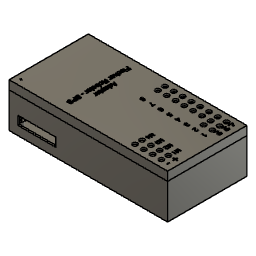
Fischer Technik v16 (Autodesk Fusion 360 design; units mm, degrees)
Autodesk Fusion 360 part; units mm, degrees
sketch "Skizze1" plane through (0, 0, 0) normal (0, 1, 0) x (1, 0, 0)
  line L0 (0, 0) -> (180, 0)
  line L1 (180, 0) -> (180, 90)
  line L2 (180, 90) -> (0, 90)
  line L3 (0, 90) -> (0, 0)
  constraint horizontal L0
  constraint vertical L1
  constraint horizontal L2
  constraint vertical L3
  constraint coincident L0.start L3.end
extrude "Extrusion1" add sketch "Skizze1" along normal blind 30 makes body 1
extrude "Extrusion2" add 1 faces at (60, 30, -60) along direction (0, 1, 0) blind 20 on bodies 1 bodies 1
ref_plane "Arbeitsebene1" through (90, 40, -45) normal (0, 1, 0) x (0, 0, 1)
split "Teilen1" by plane through (90, 40, -45) normal (0, 1, 0) bodies 1 makes body 2 at (60, 50, -60)
shell "Schale1" thickness 2 removed faces 1 at (120, 40, -60) on bodies 1
shell "Schale2" thickness 2 removed faces 1 at (120, 40, -60) on bodies 2
sketch "Skizze4" plane through (0, 0, 0) normal (0, 1, 0) x (1, 0, 0)
  circle A0 centre (6.4995, 82.5) radius 3
  circle A1 centre (172.0121, 7) radius 3
  circle A2 centre (171.9995, 82.5) radius 3
  circle A3 centre (6.5121, 7) radius 3
  dimension "d11" = 6
  dimension "d12" = 6
  dimension "d13" = 6
  dimension "d14" = 6
  dimension "d117" = 165.5
  dimension "d118" = 165.5
  dimension "d119" = 75.5
  dimension "d120" = 75.5
  measures "d11" diameter of A0
  measures "d12" diameter of A1
  measures "d13" diameter of A2
  measures "d14" diameter of A3
  measures "d117" horizontal distance of A0.centre A2.centre
  measures "d118" distance of A1.centre A3.centre
  measures "d119" vertical distance of A0.centre A3.centre
  measures "d120" vertical distance of A1.centre A2.centre
extrude "Extrusion4" add sketch "Skizze4" along normal blind 10 separate body contours A3 makes body 3
extrude "Extrusion5" add sketch "Skizze4" along normal blind 10 separate body contours A1 makes body 4
extrude "Extrusion6" add sketch "Skizze4" along normal blind 10 separate body contours A0 makes body 5
extrude "Extrusion7" add sketch "Skizze4" along normal blind 10 separate body contours A2 makes body 6
sketch "Skizze6" plane through (0, 0, 0) normal (-1, 0, 0) x (0, 0, 1)
  line L0 (0, 40) -> (-90, 40)
  line L1 (-90, 40) -> (-90, 0)
  line L2 (-90, 0) -> (0, 0)
  line L3 (0, 0) -> (0, 40)
  line L4 (-79.5, 20) -> (-10.5, 20)
  line L5 (-10.5, 20) -> (-10.5, 10.0586)
  line L6 (-10.5, 10.0586) -> (-79.5, 10.0586)
  line L7 (-79.5, 10.0586) -> (-79.5, 20)
  dimension "d24" = 69
  constraint horizontal L4
  constraint vertical L5
  constraint horizontal L6
  constraint vertical L7
  measures "d24" distance of L4.start L4.end
extrude "Extrusion8" cut sketch "Skizze6" against normal blind 2 contours L4 L5 L6 L7 bodies 1
sketch "Skizze7" plane through (0, 0, 0) normal (0, 0, 1) x (1, 0, 0)
  line L0 (180, 40) -> (0, 40)
  line L1 (0, 40) -> (0, 0)
  line L2 (0, 0) -> (180, 0)
  line L3 (180, 0) -> (180, 40)
  line L4 (10, 0) -> (53, 0)
  line L5 (53, 0) -> (53, 20)
  line L6 (53, 20) -> (10, 20)
  line L7 (10, 20) -> (10, 0)
  line L8 (10, 20) -> (53, 20)
  line L9 (53, 20) -> (53, 10)
  line L10 (53, 10) -> (10, 10)
  line L11 (10, 10) -> (10, 20)
  dimension "d27" = 43
  dimension "d123" = 10
  constraint horizontal L4
  constraint vertical L5
  constraint horizontal L6
  constraint vertical L7
  constraint coincident L2 L4.start
  constraint horizontal L8
  constraint vertical L9
  constraint horizontal L10
  constraint vertical L11
  constraint midpoint L5 L9.end
  measures "d27" distance of L4.start L4.end
  measures "d123" distance of L1 L7
sketch "Skizze8" plane through (0, 50, 0) normal (0, 1, 0) x (-1, 0, 0)
  line L0 (0, -90) -> (0, 0)
  line L1 (0, 0) -> (-180, 0)
  line L2 (-180, 0) -> (-180, -90)
  line L3 (-180, -90) -> (0, -90)
  point P0 (-165, -82)
  point P1 (-165, -74)
  point P2 (-165, -66)
  point P3 (-155, -82)
  point P4 (-155, -74)
  point P5 (-155, -66)
  point P6 (-145, -82)
  point P7 (-145, -74)
  point P8 (-135, -82)
  point P9 (-135, -74)
  point P10 (-95, -82)
  point P11 (-125, -82)
  point P12 (-115, -82)
  point P13 (-105, -82)
  point P14 (-95, -74)
  point P15 (-125, -74)
  point P16 (-115, -74)
  point P17 (-105, -74)
  dimension "d30" = 8
  dimension "d31" = 8
  dimension "d32" = 8
  dimension "d33" = 10
  dimension "d34" = 10
  dimension "d35" = 15
  dimension "d37" = 10
  dimension "d38" = 10
  dimension "d39" = 10
  dimension "d40" = 10
  dimension "d41" = 10
  constraint vertical P0 P1
  constraint vertical P1 P2
  constraint vertical P3 P4
  constraint vertical P4 P5
  constraint vertical P6 P7
  constraint vertical P8 P9
  constraint vertical P10 P14
  constraint vertical P11 P15
  constraint vertical P12 P16
  constraint vertical P13 P17
  constraint horizontal P0 P3
  constraint horizontal P6 P8
  constraint horizontal P10 P11
  constraint horizontal P12 P13
  constraint horizontal P1 P4
  constraint horizontal P7 P9
  constraint horizontal P14 P15
  constraint horizontal P16 P17
  constraint horizontal P15 P16
  constraint horizontal P9 P14
  constraint horizontal P4 P7
  constraint horizontal P2 P5
  constraint horizontal P3 P6
  constraint horizontal P8 P10
  constraint horizontal P11 P12
  measures "d30" distance of P0 P1
  measures "d31" distance of P1 P2
  measures "d32" distance of L3 P0
  measures "d33" distance of P0 P3
  measures "d34" distance of P3 P6
  measures "d35" distance of L2 P0
  measures "d37" distance of P6 P8
  measures "d38" distance of P8 P11
  measures "d39" distance of P11 P12
  measures "d40" distance of P12 P13
  measures "d41" distance of P10 P13
sketch "Skizze9" plane through (0, 50, 0) normal (0, 1, 0) x (-1, 0, 0)
  line L0 (0, 0) -> (-180, 0)
  point P0 (-165, -16)
  point P1 (-165, -8)
  point P2 (-155, -16)
  point P3 (-155, -8)
  point P4 (-145, -16)
  point P5 (-145, -8)
  point P6 (-135, -16)
  point P7 (-135, -8)
  point P8 (-165, -66)
  point P9 (-135, -74)
  point P10 (-145, -74)
  point P11 (-155, -66)
  dimension "d42" = 8
  dimension "d43" = 8
  constraint vertical P0 P1
  constraint vertical P2 P3
  constraint vertical P4 P5
  constraint vertical P6 P7
  constraint horizontal P0 P2
  constraint horizontal P4 P6
  constraint horizontal P1 P3
  constraint horizontal P5 P7
  constraint vertical P0 P8
  constraint vertical P6 P9
  constraint vertical P4 P10
  constraint vertical P2 P11
  constraint horizontal P2 P4
  constraint horizontal P1 P7
  measures "d42" distance of P1 L0
  measures "d43" distance of P0 P1
hole "Bohrung1" at (165, 50, -82) at (165, 50, -74) at (165, 50, -66) at (155, 50, -82) at (155, 50, -74) at (155, 50, -66) at (165, 50, -16) at (165, 50, -8) at (155, 50, -16) at (155, 50, -8) at (145, 50, -8) at (145, 50, -16) at (135, 50, -16) at (135, 50, -8) at (145, 50, -82) at (145, 50, -74) at (135, 50, -82) at (135, 50, -74) at (125, 50, -82) at (125, 50, -74) at (115, 50, -82) at (105, 50, -82) at (95, 50, -82) at (115, 50, -74) at (105, 50, -74) at (95, 50, -74) direction (0, -1, 0) diameter 5.5 depth 2 tip angle 180 bodies 2
sketch "Skizze10" plane through (0, 50, 0) normal (0, 1, 0) x (-1, 0, 0)
  circle A0 centre (-105, -74) radius 2.75
  circle A1 centre (-95, -82) radius 2.75
  circle A2 centre (-115, -82) radius 2.75
  circle A3 centre (-125, -82) radius 2.75
  circle A4 centre (-135, -82) radius 2.75
  circle A5 centre (-145, -82) radius 2.75
  circle A6 centre (-135, -16) radius 2.75
  circle A7 centre (-145, -8) radius 2.75
  circle A8 centre (-155, -16) radius 2.75
  circle A9 centre (-165, -16) radius 2.75
  circle A10 centre (-155, -74) radius 2.75
  circle A11 centre (-165, -66) radius 2.75
  circle A12 centre (-165, -82) radius 2.75
  circle A13 centre (-165, -74) radius 2.75
  circle A14 centre (-155, -82) radius 2.75
  circle A15 centre (-155, -66) radius 2.75
  circle A16 centre (-165, -8) radius 2.75
  circle A17 centre (-155, -8) radius 2.75
  circle A18 centre (-145, -16) radius 2.75
  circle A19 centre (-135, -8) radius 2.75
  circle A20 centre (-145, -74) radius 2.75
  circle A21 centre (-135, -74) radius 2.75
  circle A22 centre (-125, -74) radius 2.75
  circle A23 centre (-105, -82) radius 2.75
  circle A24 centre (-115, -74) radius 2.75
  circle A25 centre (-95, -74) radius 2.75
  line L0 (0, -90) -> (0, 0)
  line L1 (0, 0) -> (-180, 0)
  line L2 (-180, 0) -> (-180, -90)
  line L3 (-180, -90) -> (0, -90)
  line L4 (-171.0364, -76.774) -> (-170.9517, -76.7754) construction
  line L5 (-170.9517, -76.7754) -> (-170.8917, -73.1568) construction
  line L6 (-170.8917, -73.1568) -> (-170.9764, -73.1554) construction
  line L7 (-170.9764, -73.1554) -> (-171.0364, -76.774) construction
  line L8 (-171.0447, -69.2672) -> (-170.9608, -69.2686) construction
  line L9 (-170.9608, -69.2686) -> (-170.8838, -64.656) construction
  line L10 (-170.8838, -64.656) -> (-170.9677, -64.6546) construction
  line L11 (-170.9677, -64.6546) -> (-171.0447, -69.2672) construction
  line L12 (-162.4935, -58.9995) -> (-162.4944, -54.6405) construction
  line L13 (-162.4944, -54.6405) -> (-167.5074, -54.6415) construction
  line L14 (-167.5074, -54.6415) -> (-167.5065, -59.0005) construction
  line L15 (-167.5065, -59.0005) -> (-162.4935, -58.9995) construction
  line L16 (-152.495, -59.6156) -> (-152.4933, -54.0295) construction
  line L17 (-152.4933, -54.0295) -> (-157.5033, -54.028) construction
  line L18 (-157.5033, -54.028) -> (-157.505, -59.6141) construction
  line L19 (-157.505, -59.6141) -> (-152.495, -59.6156) construction
  line L20 (-142.5028, -60.1186) -> (-142.4948, -53.5355) construction
  line L21 (-142.4948, -53.5355) -> (-147.4893, -53.5295) construction
  line L22 (-147.4893, -53.5295) -> (-147.4972, -60.1126) construction
  line L23 (-147.4972, -60.1126) -> (-142.5028, -60.1186) construction
  line L24 (-132.5014, -60.1298) -> (-132.5029, -53.51) construction
  line L25 (-132.5029, -53.51) -> (-137.5001, -53.5111) construction
  line L26 (-137.5001, -53.5111) -> (-137.4986, -60.1309) construction
  line L27 (-137.4986, -60.1309) -> (-132.5014, -60.1298) construction
  line L28 (-122.0178, -60.1305) -> (-121.9983, -53.5468) construction
  line L29 (-121.9983, -53.5468) -> (-127.9627, -53.5292) construction
  line L30 (-127.9627, -53.5292) -> (-127.9822, -60.1129) construction
  line L31 (-127.9822, -60.1129) -> (-122.0178, -60.1305) construction
  line L32 (-112.0324, -60.6387) -> (-111.9975, -53.0581) construction
  line L33 (-111.9975, -53.0581) -> (-117.9326, -53.0307) construction
  line L34 (-117.9326, -53.0307) -> (-117.9676, -60.6113) construction
  line L35 (-117.9676, -60.6113) -> (-112.0324, -60.6387) construction
  line L36 (-162.5074, -26.261) -> (-162.5038, -23.0028) construction
  line L37 (-162.5038, -23.0028) -> (-167.4962, -22.9972) construction
  line L38 (-167.4962, -22.9972) -> (-167.4998, -26.2555) construction
  line L39 (-167.4998, -26.2555) -> (-162.5074, -26.261) construction
  line L40 (-142.0105, -27.6502) -> (-142.0044, -21.6148) construction
  line L41 (-142.0044, -21.6148) -> (-147.9956, -21.6087) construction
  line L42 (-147.9956, -21.6087) -> (-148.0018, -27.6441) construction
  line L43 (-148.0018, -27.6441) -> (-142.0105, -27.6502) construction
  line L44 (-151.9984, -29.1437) -> (-151.9995, -20.1075) construction
  line L45 (-151.9995, -20.1075) -> (-158.0005, -20.1083) construction
  line L46 (-158.0005, -20.1083) -> (-157.9994, -29.1445) construction
  line L47 (-157.9994, -29.1445) -> (-151.9984, -29.1437) construction
  line L48 (-132.512, -27.6497) -> (-132.505, -21.6146) construction
  line L49 (-132.505, -21.6146) -> (-137.495, -21.6088) construction
  line L50 (-137.495, -21.6088) -> (-137.502, -27.6439) construction
  line L51 (-137.502, -27.6439) -> (-132.512, -27.6497) construction
  line L52 (-169.8709, -84.3652) -> (-166.7741, -84.3566) construction
  line L53 (-166.7741, -84.3566) -> (-166.7871, -79.6263) construction
  line L54 (-166.7871, -79.6263) -> (-169.884, -79.6348) construction
  line L55 (-169.884, -79.6348) -> (-169.8709, -84.3652) construction
  line L56 (-101.5, -61.8325) -> (-101.5, -51.8096) construction
  line L57 (-101.5, -51.8096) -> (-108.5, -51.8096) construction
  line L58 (-108.5, -51.8096) -> (-108.5, -61.8325) construction
  line L59 (-108.5, -61.8325) -> (-101.5, -61.8325) construction
  line L60 (-92.065, -62.0835) -> (-92.065, -51.5586) construction
  line L61 (-92.065, -51.5586) -> (-97.935, -51.5586) construction
  line L62 (-97.935, -51.5586) -> (-97.935, -62.0835) construction
  line L63 (-97.935, -62.0835) -> (-92.065, -62.0835) construction
  line L64 (-169.7376, -19.25) -> (-169.7376, -12.75) construction
  line L65 (-169.7376, -12.75) -> (-174.2376, -12.75) construction
  line L66 (-174.2376, -12.75) -> (-174.2376, -19.25) construction
  line L67 (-174.2376, -19.25) -> (-169.7376, -19.25) construction
  line L68 (-168.75, -11.2496) -> (-168.75, -4.7504) construction
  line L69 (-168.75, -4.7504) -> (-174.3763, -4.7504) construction
  line L70 (-174.3763, -4.7504) -> (-174.3763, -11.2496) construction
  line L71 (-174.3763, -11.2496) -> (-168.75, -11.2496) construction
  point P0 (-165, -66)
  point P1 (-155, -66)
  point P2 (-145, -74)
  point P3 (-135, -74)
  point P4 (-165, -16)
  point P5 (-155, -16)
  point P6 (-145, -16)
  point P7 (-135, -16)
  point P8 (-165, -8)
  dimension "d48" = 4
  dimension "d49" = 4
  dimension "d50" = 5
  dimension "d51" = 5
  dimension "d52" = 5
  dimension "d53" = 5
  dimension "d54" = 5
  dimension "d55" = 5
  dimension "d60" = 4
  dimension "d61" = 4
  dimension "d62" = 4
  dimension "d63" = 4
  dimension "d65" = 7
  dimension "d66" = 7
  dimension "d110" = 6
  dimension "d111" = 6
  dimension "d124" = 5
  dimension "d127" = 5
  dimension "d128" = 5
  dimension "d129" = 7
  dimension "d130" = 7
  text T0 "9V" font "Arial" height 4 align centre top in box 0.0847 x 3.6191 at (-171.0364, -76.774) x (0.999863, -0.016561) y (0.016561, 0.999863) spacing 1 kerned
  text T1 "0V" font "Arial" height 4 align centre top in box 0.0839 x 4.6133 at (-171.0447, -69.2672) x (0.999861, -0.01669) y (0.01669, 0.999861) spacing 1 kerned
  text T2 "1" font "Arial" height 5 align centre top in box 4.359 x 5.0129 at (-162.4935, -58.9995) x (-0.000209, 1) y (-1, -0.000209) spacing 1 kerned
  text T3 "2" font "Arial" height 5 align centre top in box 5.5861 x 5.01 at (-152.495, -59.6156) x (0.00031, 1) y (-1, 0.00031) spacing 1 kerned
  text T4 "3\n" font "Arial" height 5 align centre top in box 6.5831 x 4.9945 at (-142.5028, -60.1186) x (0.001213, 0.999999) y (-0.999999, 0.001213) spacing 1 kerned
  text T5 "4" font "Arial" height 5 align centre top in box 6.6198 x 4.9972 at (-132.5014, -60.1298) x (-0.000226, 1) y (-1, -0.000226) spacing 1 kerned
  text T6 "5" font "Arial" height 5 align centre top in box 6.5838 x 5.9644 at (-122.0178, -60.1305) x (0.002958, 0.999996) y (-0.999996, 0.002958) spacing 1 kerned
  text T7 "6" font "Arial" height 5 align centre top in box 7.5807 x 5.9352 at (-112.0324, -60.6387) x (0.004609, 0.999989) y (-0.999989, 0.004609) spacing 1 kerned
  text T8 "M1" font "Arial" height 4 align centre top in box 3.2583 x 4.9924 at (-162.5074, -26.261) x (0.001108, 0.999999) y (-0.999999, 0.001108) spacing 1 kerned
  text T9 "M3" font "Arial" height 4 align centre top in box 6.0354 x 5.9913 at (-142.0105, -27.6502) x (0.001018, 0.999999) y (-0.999999, 0.001018) spacing 1 kerned
  text T10 "M2" font "Arial" height 4 align centre top in box 9.0362 x 6.001 at (-151.9984, -29.1437) x (-0.000121, 1) y (-1, -0.000121) spacing 1 kerned
  text T11 "M4" font "Arial" height 4 align centre top in box 6.0351 x 4.99 at (-132.512, -27.6497) x (0.001164, 0.999999) y (-0.999999, 0.001164) spacing 1 kerned
  text T12 "I" font "Arial" height 5 align left top in box 3.0969 x 4.7304 at (-169.8709, -84.3652) x (0.999996, 0.002757) y (-0.002757, 0.999996) spacing 1 kerned
  text T13 "7" font "Arial" height 5 align centre middle in box 10.0229 x 7 at (-101.5, -61.8325) x (0, 1) y (-1, 0) spacing 1 kerned
  text T14 "8" font "Arial" height 5 align centre middle in box 10.5249 x 5.87 at (-92.065, -62.0835) x (0, 1) y (-1, 0) spacing 1 kerned
  text T15 "+" font "Arial" height 7 align centre middle in box 6.5 x 4.5 at (-169.7376, -19.25) x (0, 1) y (-1, 0) spacing 1 kerned
  text T16 "-" font "Arial" height 7 align centre middle in box 6.4992 x 5.6263 at (-168.75, -11.2496) x (0, 1) y (-1, 0) spacing 1 kerned
  constraint vertical P0
  constraint vertical P1
  constraint vertical P2
  constraint vertical P3
  constraint vertical A22.centre
  constraint vertical A24.centre
  constraint vertical P4
  constraint vertical P5
  constraint vertical P6
  constraint vertical P7
  constraint horizontal A12.centre
  constraint vertical A0.centre
  constraint vertical A25.centre
  constraint horizontal P4
  constraint horizontal P8
  measures "d65" distance of P4
  measures "d66" distance of P0
  measures "d110" distance of P0
  measures "d111" distance of A13.centre
combine "Kombinieren1" operation add target body 1 tool bodies 3 4 5 6
hole "Bohrung2" at (6.5121, 10, -7) direction (0, -1, 0) diameter 1.9 depth 7 tip angle 180 bodies 1
hole "Bohrung3" at (6.4995, 10, -82.5) direction (0, -1, 0) diameter 1.9 depth 7 tip angle 180 bodies 1
hole "Bohrung4" at (171.9995, 10, -82.5) direction (0, -1, 0) diameter 1.9 depth 7 tip angle 180 bodies 1
hole "Bohrung5" at (172.0121, 10, -7) direction (0, -1, 0) diameter 1.9 depth 7 tip angle 180 bodies 1
extrude "Extrusion12" cut sketch "Skizze7" against normal blind 1 contours L5 L6 L7 L8 L9 L10 L11 bodies 1
sketch "Skizze11" plane through (0, 50, 0) normal (0, 1, 0) x (-1, 0, 0)
  line L0 (0, -90) -> (0, 0)
  line L1 (0, 0) -> (-180, 0)
  line L2 (-180, 0) -> (-180, -90)
  line L3 (-180, -90) -> (0, -90)
  circle A0 centre (-95, -74) radius 2.75
  circle A1 centre (-115, -74) radius 2.75
  circle A2 centre (-105, -82) radius 2.75
  circle A3 centre (-125, -74) radius 2.75
  circle A4 centre (-135, -74) radius 2.75
  circle A5 centre (-145, -74) radius 2.75
  circle A6 centre (-135, -8) radius 2.75
  circle A7 centre (-145, -16) radius 2.75
  circle A8 centre (-155, -8) radius 2.75
  circle A9 centre (-165, -8) radius 2.75
  circle A10 centre (-155, -66) radius 2.75
  circle A11 centre (-155, -82) radius 2.75
  circle A12 centre (-165, -74) radius 2.75
  circle A13 centre (-165, -66) radius 2.75
  circle A14 centre (-155, -74) radius 2.75
  circle A15 centre (-155, -16) radius 2.75
  circle A16 centre (-145, -8) radius 2.75
  circle A17 centre (-135, -16) radius 2.75
  circle A18 centre (-145, -82) radius 2.75
  circle A19 centre (-135, -82) radius 2.75
  circle A20 centre (-125, -82) radius 2.75
  circle A21 centre (-115, -82) radius 2.75
  circle A22 centre (-95, -82) radius 2.75
  circle A23 centre (-105, -74) radius 2.75
  circle A24 centre (-165, -82) radius 2.75
  circle A25 centre (-165, -16) radius 2.75
  point P0 (-6.5, -7)
  point P1 (-172, -82.5)
extrude "Extrusion24" cut 1 faces at (24.3333, 13.3333, -1) along direction (0, 0, -1) blind 5 on bodies 1 bodies 1
hole "Bohrung6" at (172, 50, -82.5) at (6.5, 50, -7) direction (0, -1, 0) diameter 2 depth 5 tip angle 180 bodies 2
sketch "Skizze12" plane through (0, 40, 0) normal (0, 1, 0) x (-1, 0, 0)
  line L0 (-178, -2) -> (-2, -2)
  line L1 (-2, -2) -> (-2, -88)
  line L2 (-2, -88) -> (-178, -88)
  line L3 (-178, -88) -> (-178, -2)
  line L4 (-180, -90) -> (0, -90)
  line L5 (0, -90) -> (0, 0)
  line L6 (0, 0) -> (-180, 0)
  line L7 (-180, 0) -> (-180, -90)
sketch "Skizze15" plane through (0, 40, 0) normal (0, 1, 0) x (-1, 0, 0)
  line L0 (-2, -2) -> (-178, -2)
  line L1 (-178, -2) -> (-178, -88)
  line L2 (-178, -88) -> (-2, -88)
  line L3 (-2, -88) -> (-2, -2)
  line L4 (-180, 0) -> (-180, -90)
  line L5 (0, -10.5) -> (0, -79.5)
  line L6 (0, 0) -> (-180, 0)
  line L7 (-180, -90) -> (0, -90)
  dimension "d140" = 2
  dimension "d141" = 2
  dimension "d142" = 2
  dimension "d143" = 2
  constraint horizontal L0
  constraint vertical L1
  constraint horizontal L2
  constraint vertical L3
  measures "d140" distance of L1 L4
  measures "d141" distance of L3 L5
  measures "d142" distance of L0 L6
  measures "d143" distance of L2 L7
extrude "Extrusion15" add sketch "Skizze12" along normal blind 4 contours L0 L1 L2 L3 bodies 2
extrude "Extrusion16" add sketch "Skizze15" against normal blind 3 bodies 2
sketch "Skizze3" plane through (0, 0, 0) normal (0, 1, 0) x (1, 0, 0)
  circle A0 centre (180, -30) radius 3
  dimension "d8" = 6
  measures "d8" diameter of A0
extrude "Extrusion17" add 1 faces at (119.3333, 37, -30.6667) along direction (0, -1, 0) blind 2 on bodies 2 bodies 2
sketch "Skizze17" plane through (0, 35, 0) normal (0, -1, 0) x (1, 0, 0)
  line L0 (2, -2) -> (2, -88)
  line L1 (2, -88) -> (178, -88)
  line L2 (178, -88) -> (178, -2)
  line L3 (178, -2) -> (2, -2)
  line L4 (3.5, -3.5) -> (176.5, -3.5)
  line L5 (176.5, -3.5) -> (176.5, -86.5)
  line L6 (176.5, -86.5) -> (3.5, -86.5)
  line L7 (3.5, -86.5) -> (3.5, -3.5)
  dimension "d103" = 1.5
  dimension "d104" = 1.5
  dimension "d105" = 1.5
  dimension "d106" = 1.5
  constraint horizontal L4
  constraint vertical L5
  constraint horizontal L6
  constraint vertical L7
  measures "d103" distance of L3 L4
  measures "d104" distance of L1 L6
  measures "d105" distance of L2 L5
  measures "d106" distance of L0 L7
extrude "Extrusion18" cut sketch "Skizze17" against normal blind 10 contours L4 L5 L6 L7 bodies 2
sketch "Skizze18" plane through (0, 50, 0) normal (0, 1, 0) x (-1, 0, 0)
  line L0 (-46.2864, -86.6174) -> (-46.3071, -4.1466) construction
  line L1 (-46.3071, -4.1466) -> (-74.057, -4.1536) construction
  line L2 (-74.057, -4.1536) -> (-74.0362, -86.6243) construction
  line L3 (-74.0362, -86.6243) -> (-46.2864, -86.6174) construction
  dimension "d114" = 5
  text T0 "Adapter\nFischer Roboter - SPS" font "Arial" height 5 align centre middle in box 82.4707 x 27.7499 at (-46.2864, -86.6174) x (-0.000251, 1) y (-1, -0.000251) spacing 1 kerned
extrude "Extrusion19" cut sketch "Skizze18" against normal blind 0.5 text T0 bodies 2
extrude "Extrusion22" cut sketch "Skizze10" against normal blind 1 text T12 T0 T1 T2 T3 T4 T5 T6 T7 T13 T14 T15 T16 T8 T10 T9 T11 bodies 2
